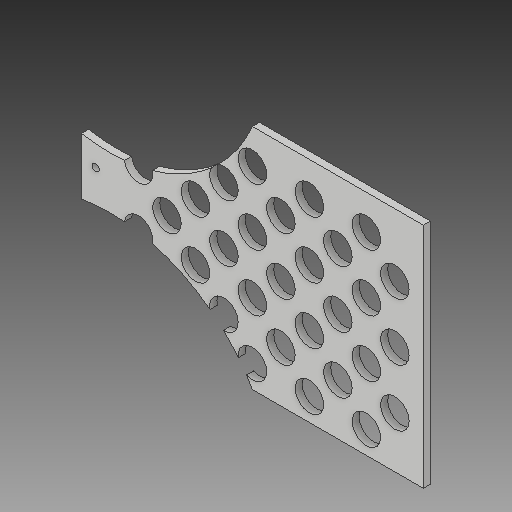
# Autodesk Inventor part: FlapperSlapperPlate
Saved by Autodesk Inventor 2019 (Build 230136000, 136)
## iProperties
Created: 2018-01-13
Part Number: FlapperSlapperPlate
Material: Generic
Document SubType Name: Modeling
Designer: User
Density: 1 g/cm^3
Appearance: Default
Mass: 23.4463 g
Surface Area: 196.204 cm^2
Volume: 23.4463 cm^3
Author: User
Autodesk Inventor part; units mm, degrees
ref_plane "YZ Plane" through (0, 0, 0) normal (1, 0, 0) x (0, 1, 0)
ref_plane "XZ Plane" through (0, 0, 0) normal (0, 1, 0) x (-1, 0, 0)
ref_plane "XY Plane" through (0, 0, 0) normal (0, 0, 1) x (1, 0, 0)
sketch "Sketch1" plane through (0, 0, 0) normal (0, 0, 1) x (1, 0, 0)
  line L0 (0, 0) -> (152.4, 0)
  line L1 (152.4, 0) -> (152.4, -101.6)
  line L2 (152.4, -101.6) -> (0, -101.6)
  line L3 (0, -101.6) -> (0, 0)
  dimension "d0" = 152.4
  dimension "d1" = 101.6
  constraints: 8 end point, 2 parallel, 1 horizontal, 1 perpendicular
  measures "d0" distance of L1.end L2.end
  measures "d1" distance of L0.end L1.end
extrude "Extrusion1" add sketch "Sketch1" along normal blind 3.175
sketch "Sketch2" plane through (0, 0, 3.175) normal (0, 0, 1) x (1, 0, 0)
  line L0 (0, 0) -> (0, -101.6) projected
  line L1 (152.4, 0) -> (0, 0) projected
  line L2 (152.4, -101.6) -> (152.4, 0) projected
  line L3 (0, -101.6) -> (152.4, -101.6) projected
  line L4 (25.4, -91.5497) -> (50.8, -91.5497)
  line L5 (50.8, -91.5497) -> (50.8, -66.1497)
  line L6 (50.8, -66.1497) -> (25.4, -66.1497)
  line L7 (25.4, -66.1497) -> (25.4, -91.5497)
  point P0 (76.2, -91.5497)
  point P1 (101.6, -91.5497)
  point P2 (127, -91.5497)
  point P3 (76.2, -66.1497)
  point P4 (101.6, -66.1497)
  point P5 (127, -66.1497)
  point P6 (25.4, -40.7497)
  point P7 (50.8, -40.7497)
  point P8 (76.2, -40.7497)
  point P9 (101.6, -40.7497)
  point P10 (127, -40.7497)
  point P11 (25.4, -15.3497)
  point P12 (50.8, -15.3497)
  point P13 (76.2, -15.3497)
  point P14 (101.6, -15.3497)
  point P15 (127, -15.3497)
  point P16 (38.1, -78.8497)
  point P17 (63.5, -78.8497)
  point P18 (88.9, -78.8497)
  point P19 (114.3, -78.8497)
  point P20 (139.7, -78.8497)
  point P21 (38.1, -53.4497)
  point P22 (63.5, -53.4497)
  point P23 (88.9, -53.4497)
  point P24 (114.3, -53.4497)
  point P25 (139.7, -53.4497)
  point P26 (38.1, -28.0497)
  point P27 (63.5, -28.0497)
  point P28 (88.9, -28.0497)
  point P29 (114.3, -28.0497)
  point P30 (139.7, -28.0497)
  dimension "d5" = 25.4
  dimension "d8" = 25.4
  dimension "d11" = 25.4
  dimension "d16" = 25.4
  dimension "d19" = 25.4
  constraints: 8 end point, 3 horizontal, 2 parallel, 2 vertical, 1 perpendicular, 33 other
  measures "d5" distance from line of L0 L4.start
  measures "d8" distance of L4.start point (50.8, -91.55)
  measures "d11" distance of L4.start point (25.4, -66.15)
  measures "d16" distance of point (38.1, -78.85) point (63.5, -78.85)
  measures "d19" distance of point (38.1, -78.85) point (38.1, -53.45)
hole "Hole1" at (25.4, -91.5497, 3.175) at (50.8, -91.5497, 3.175) at (76.2, -91.5497, 3.175) at (101.6, -91.5497, 3.175) at (127, -91.5497, 3.175) at (25.4, -66.1497, 3.175) at (50.8, -66.1497, 3.175) at (76.2, -66.1497, 3.175) at (101.6, -66.1497, 3.175) at (127, -66.1497, 3.175) at (25.4, -40.7497, 3.175) at (50.8, -40.7497, 3.175) at (76.2, -40.7497, 3.175) at (101.6, -40.7497, 3.175) at (127, -40.7497, 3.175) at (25.4, -15.3497, 3.175) at (50.8, -15.3497, 3.175) at (76.2, -15.3497, 3.175) at (101.6, -15.3497, 3.175) at (127, -15.3497, 3.175) at (38.1, -78.8497, 3.175) at (63.5, -78.8497, 3.175) at (88.9, -78.8497, 3.175) at (114.3, -78.8497, 3.175) at (139.7, -78.8497, 3.175) at (38.1, -53.4497, 3.175) at (63.5, -53.4497, 3.175) at (88.9, -53.4497, 3.175) at (114.3, -53.4497, 3.175) at (139.7, -53.4497, 3.175) at (38.1, -28.0497, 3.175) at (63.5, -28.0497, 3.175) at (88.9, -28.0497, 3.175) at (114.3, -28.0497, 3.175) at (139.7, -28.0497, 3.175) direction (0, 0, -1) diameter 12.7 depth 25.4 tip angle 118
sketch "Sketch3" plane through (0, 0, 3.175) normal (0, 0, 1) x (1, 0, 0)
  line L0 (0, 0) -> (0, -101.6) projected
  line L1 (0, -50.8) -> (6.35, -50.8)
  dimension "d29" = 6.35
  dimension "d39" = 101.6
  constraints: 2 end point, 1 coincident, 1 horizontal, 1 midpoint
  measures "d29" distance of L1.start L1.end
  measures "d39" distance of L0.start L0.end
hole "Hole2" at (6.35, -50.8, 3.175) direction (0, 0, -1) diameter 3.175 depth 25.4 tip angle 118
sketch "Sketch4" plane through (0, 0, 3.175) normal (0, 0, 1) x (1, 0, 0)
  circle A0 centre (6.35, -50.8) radius 1.5875 projected
  circle A1 centre (114.3, -28.0497) radius 6.35 projected
  circle A2 centre (63.5, -28.0497) radius 6.35 projected
  circle A3 centre (139.7, -53.4497) radius 6.35 projected
  circle A4 centre (88.9, -53.4497) radius 6.35 projected
  circle A5 centre (38.1, -53.4497) radius 6.35 projected
  circle A6 centre (114.3, -78.8497) radius 6.35 projected
  circle A7 centre (63.5, -78.8497) radius 6.35 projected
  circle A8 centre (127, -15.3497) radius 6.35 projected
  circle A9 centre (76.2, -15.3497) radius 6.35 projected
  circle A10 centre (25.4, -15.3497) radius 6.35 projected
  circle A11 centre (101.6, -40.7497) radius 6.35 projected
  circle A12 centre (50.8, -40.7497) radius 6.35 projected
  circle A13 centre (127, -66.1497) radius 6.35 projected
  circle A14 centre (76.2, -66.1497) radius 6.35 projected
  circle A15 centre (25.4, -66.1497) radius 6.35 projected
  circle A16 centre (101.6, -91.5497) radius 6.35 projected
  circle A17 centre (50.8, -91.5497) radius 6.35 projected
  circle A18 centre (25.4, -91.5497) radius 6.35 projected
  circle A19 centre (76.2, -91.5497) radius 6.35 projected
  circle A20 centre (127, -91.5497) radius 6.35 projected
  circle A21 centre (50.8, -66.1497) radius 6.35 projected
  circle A22 centre (101.6, -66.1497) radius 6.35 projected
  circle A23 centre (25.4, -40.7497) radius 6.35 projected
  circle A24 centre (76.2, -40.7497) radius 6.35 projected
  circle A25 centre (127, -40.7497) radius 6.35 projected
  circle A26 centre (50.8, -15.3497) radius 6.35 projected
  circle A27 centre (101.6, -15.3497) radius 6.35 projected
  circle A28 centre (38.1, -78.8497) radius 6.35 projected
  circle A29 centre (88.9, -78.8497) radius 6.35 projected
  circle A30 centre (139.7, -78.8497) radius 6.35 projected
  circle A31 centre (63.5, -53.4497) radius 6.35 projected
  circle A32 centre (114.3, -53.4497) radius 6.35 projected
  circle A33 centre (38.1, -28.0497) radius 6.35 projected
  circle A34 centre (88.9, -28.0497) radius 6.35 projected
  circle A35 centre (139.7, -28.0497) radius 6.35 projected
  line L0 (152.4, 0) -> (0, 0) projected
  line L1 (0, 0) -> (0, -101.6) projected
  line L2 (0, -101.6) -> (152.4, -101.6) projected
  line L3 (152.4, -101.6) -> (152.4, 0) projected
  line L4 (152.4, -101.6) -> (0, -101.6) projected
  line L5 (0, 0) -> (0, -101.6) projected
  circle A36 centre (25.4, -66.1497) radius 6.35 projected
  arc A37 (76.2, -101.6) -> (0, -66.1497) centre (12.7, -138.4718) ccw
  line L6 (0, 0) -> (152.4, 0) projected
  circle A38 centre (25.4, -40.7497) radius 6.35 projected
  arc A39 (0, -40.7497) -> (76.2, 0) centre (12.7, 27.122) ccw
  line L7 (76.2, -101.6) -> (0, -101.6)
  line L8 (0, -101.6) -> (0, -66.1497)
  line L9 (0, -40.7497) -> (0, 0)
  line L10 (0, 0) -> (76.2, 0)
  line L11 (76.2, 0) -> (0, 0)
  arc A40 (76.2, -101.6) -> (0, -66.1497) centre (12.7, -138.4718) ccw
  arc A41 (0, -40.7497) -> (76.2, 0) centre (12.7, 27.122) ccw
  constraints: 12 point on circle, 10 end point, 4 centre point, 4 collinear, 2 midpoint, 2 point on line
extrude "Extrusion2" cut sketch "Sketch4" against normal blind 25.4 contours A39 A2 | A2 A39 A23 L1 L0 | A39 A23 | L2 L1 A37 A15 A7 A19 | A19 A37 | A37 A15 | A7 A37 picked at (59.133, -23.6572) picked at (25.2529, -38.6166) picked at (71.5308, -94.9999) picked at (24.7885, -68.1972) picked at (60.0035, -82.9534)
body "Solid1"
